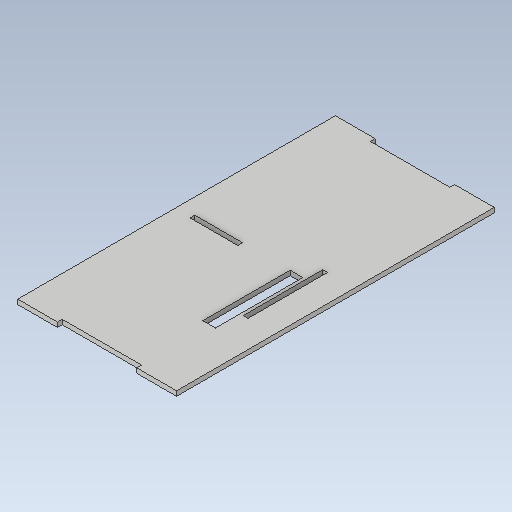
# Autodesk Inventor part: Piso
Saved by Autodesk Inventor 2020 (Build 240168000, 168)
## iProperties
Created: 2020-03-11
Part Number: Piso
Material: Genérico
Document SubType Name: Modeling
Designer: joser
Density: 1 g/cm^3
Appearance: Valor por defecto
Author: joser
Autodesk Inventor part; units mm, degrees
ref_plane "YZ Plane" through (0, 0, 0) normal (1, 0, 0) x (0, 1, 0)
ref_plane "XZ Plane" through (0, 0, 0) normal (0, 1, 0) x (-1, 0, 0)
ref_plane "XY Plane" through (0, 0, 0) normal (0, 0, 1) x (1, 0, 0)
sketch "Boceto1" plane through (0, 0, 0) normal (0, 1, 0) x (-1, 0, 0)
  line L0 (50, 100) -> (50, -100)
  line L1 (-50, 100) -> (50, -100) construction
  line L2 (50, 100) -> (-50, -100) construction
  line L3 (25, 100) -> (25, 97)
  line L4 (25, 97) -> (-25, 97)
  line L5 (-25, 97) -> (-25, 100)
  line L6 (-50, 100) -> (-25, 100)
  line L7 (25, 100) -> (50, 100)
  line L8 (25, -100) -> (25, -97)
  line L9 (25, -97) -> (-25, -97)
  line L10 (-25, -97) -> (-25, -100)
  line L11 (50, -100) -> (25, -100)
  line L12 (-25, -100) -> (-50, -100)
  line L13 (-50, -100) -> (-50, 100)
  point P0 (0, 0)
  dimension "d0" = 100
  dimension "d1" = 200
  dimension "d4" = 3
  dimension "d5" = 50
  dimension "d7" = 3
  dimension "d8" = 50
  dimension "d12" = 25
  constraints: 28 end point, 8 perpendicular, 5 parallel, 3 collinear, 2 horizontal, 2 midpoint, 2 vertical
  measures "d0" distance of L0.end L2.end
  measures "d1" distance of L0.start L0.end
  measures "d4" distance of L3.start L3.end
  measures "d5" distance of L3.end L4.end
  measures "d7" distance of L8.start L8.end
  measures "d8" distance of L8.end L9.end
  measures "d12" distance between parallel lines of L13 L5
extrude "Extrusión1" add sketch "Boceto1" along normal blind 3
sketch "Boceto2" plane through (0, 3, 0) normal (0, 1, 0) x (1, 0, 0)
  line L0 (33, 12) -> (30, 12)
  line L1 (30, 12) -> (30, -38)
  line L2 (30, -38) -> (33, -38)
  line L3 (33, -38) -> (33, 12)
  line L4 (50, 100) -> (25, 100) projected
  line L5 (-50, 100) -> (-50, -100) projected
  point P0 (0, 0)
  dimension "d17" = 3
  dimension "d18" = 50
  dimension "d19" = 88
  dimension "d20" = 80
  constraints: 8 end point, 2 parallel, 1 horizontal, 1 perpendicular
  measures "d17" distance of L2.end L1.end
  measures "d18" distance of L1.end L0.end
  measures "d19" distance between parallel lines of L4 L0
  measures "d20" distance between parallel lines of L5 L1
extrude "Extrusión2" cut sketch "Boceto2" against normal blind 3
sketch "Boceto3" plane through (0, 0, 0) normal (0, -1, 0) x (1, 0, 0)
  line L0 (-40, -1.5) -> (-10, -1.5)
  line L1 (-10, -1.5) -> (-10, 1.5)
  line L2 (-10, 1.5) -> (-40, 1.5)
  line L3 (-40, 1.5) -> (-40, -1.5)
  line L4 (-50, -100) -> (-25, -100) projected
  line L5 (30, -12) -> (30, 38) projected
  point P0 (0, 0)
  dimension "d23" = 30
  dimension "d24" = 3
  dimension "d25" = 98.5
  dimension "d26" = 40
  constraints: 8 end point, 2 parallel, 1 horizontal, 1 perpendicular
  measures "d23" distance of L2.end L1.end
  measures "d24" distance of L1.end L0.end
  measures "d25" distance between parallel lines of L4 L0
  measures "d26" distance between parallel lines of L5 L1
extrude "Extrusión3" cut sketch "Boceto3" against normal blind 3
sketch "Boceto4" plane through (0, 3, 0) normal (0, 1, 0) x (1, 0, 0)
  line L0 (28, 1.5) -> (20, 1.5)
  line L1 (20, 1.5) -> (20, -53.5)
  line L2 (20, -53.5) -> (28, -53.5)
  line L3 (28, -53.5) -> (28, 1.5)
  line L4 (-25, -97) -> (25, -97) projected
  line L5 (30, -38) -> (30, 12) projected
  line L6 (28, -26) -> (20, -26) construction
  line L7 (25, -100) -> (50, -100) projected
  point P0 (0, 0)
  dimension "d29" = 55
  dimension "d30" = 8
  dimension "d32" = 2
  dimension "d35" = 74
  constraints: 10 end point, 2 midpoint, 2 parallel, 1 horizontal, 1 perpendicular
  measures "d29" distance of L1.end L0.end
  measures "d30" distance between parallel lines of L1 L3
  measures "d32" distance between parallel lines of L5 L3
  measures "d35" distance between parallel lines of L7 L6
extrude "Extrusión4" cut sketch "Boceto4" against normal blind 3
